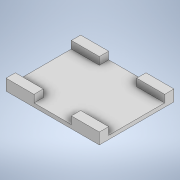
# Autodesk Inventor part: крышка кожуха нижняя
Saved by Autodesk Inventor 2020.1 (Build 241239000, 239)
## iProperties
Created: 2022-04-03
Part Number: крышка кожуха нижняя
Material: Типовые
Document SubType Name: Modeling
Designer: User
Density: 1 g/cm^3
Appearance: По умолчанию
Author: User
Autodesk Inventor part; units mm, degrees
ref_plane "YZ Plane" through (0, 0, 0) normal (1, 0, 0) x (0, 1, 0)
ref_plane "XZ Plane" through (0, 0, 0) normal (0, 1, 0) x (-1, 0, 0)
ref_plane "XY Plane" through (0, 0, 0) normal (0, 0, 1) x (1, 0, 0)
sketch "Эскиз1" plane through (0, 0, 0) normal (0, 1, 0) x (-1, 0, 0)
  line L0 (0, 0) -> (-25, 0)
  line L1 (-25, 0) -> (-25, 20)
  line L2 (-25, 20) -> (0, 20)
  line L3 (0, 20) -> (0, 0)
  dimension "d0" = 25
  dimension "d1" = 20
  constraints: 8 end point, 2 parallel, 1 horizontal, 1 perpendicular
  measures "d0" distance of L0.start L0.end
  measures "d1" distance of L2.end L0.start
extrude "Выдавливание1" add sketch "Эскиз1" along normal blind 2
sketch "Эскиз2" plane through (0, 2, 0) normal (0, 1, 0) x (1, 0, 0)
  line L0 (25, -20) -> (25, 0) projected
  line L1 (25, 0) -> (10, 0)
  line L2 (10, 0) -> (10, -5)
  line L3 (10, -5) -> (25, -5)
  line L4 (25, -5) -> (25, 0)
  point P0 (0, 0)
  dimension "d4" = 15
  dimension "d5" = 5
  constraints: 8 end point, 2 parallel, 1 horizontal, 1 perpendicular
  measures "d4" distance of L2.end L3.end
  measures "d5" distance of L1.end L2.end
extrude "Выдавливание2" add sketch "Эскиз2" along normal blind 4
mirror "Зеркальное отражение1" about plane through (0, 0, 20) normal (0, 0, 1)
mirror "Зеркальное отражение2" about plane through (0, 0, 0) normal (-1, 0, 0)
